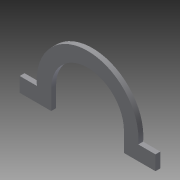
# Autodesk Inventor part: holder
Saved by Autodesk Inventor 2015 (Build 190159000, 159)
## iProperties
Created: 2014-08-30
Part Number: holder
Material: Generic
Document SubType Name: Modeling
Designer: shohei
Density: 1 g/cm^3
Appearance: Default
Author: shohei
Autodesk Inventor part; units mm, degrees
ref_plane "YZ Plane" through (0, 0, 0) normal (1, 0, 0) x (0, 1, 0)
ref_plane "XZ Plane" through (0, 0, 0) normal (0, 1, 0) x (-1, 0, 0)
ref_plane "XY Plane" through (0, 0, 0) normal (0, 0, 1) x (1, 0, 0)
sketch "Sketch1" plane through (0, 0, 0) normal (0, 1, 0) x (-1, 0, 0)
  arc A0 (104.5316, -9.9117) -> (-104.5321, -9.9065) centre (0, 0) ccw
  line L0 (104.5316, -9.9117) -> (140, -9.9117)
  line L1 (140, -9.9117) -> (140, -39.9117)
  line L2 (-140, -39.9117) -> (-140, -9.9065)
  line L3 (0, -68.8947) -> (0, 133.9861) projected
  line L4 (135.3627, -9.9117) -> (104.5316, -9.9117)
  line L5 (-104.5321, -9.9065) -> (-140, -9.9065)
  line L6 (74.3541, -9.8216) -> (74.3541, -9.9117)
  line L7 (74.3541, -9.8216) -> (74.3541, -9.9117)
  line L8 (140, -39.9117) -> (75, -39.9117)
  line L9 (-75, -39.9117) -> (-140, -39.9117)
  line L10 (-196, 0) -> (196, 0) projected
  arc A1 (74.3429, -9.9065) -> (74.3541, -9.8216) centre (0, 0) ccw
  arc A2 (75, 0) -> (-75, 0) centre (0, 0) ccw
  line L11 (75, 0) -> (75, -39.9117)
  line L12 (-75, -39.9117) -> (-75, 0)
  dimension "d3" = 30
  dimension "d4" = 280
  dimension "d5" = 140
  constraints: 22 end point, 9 perpendicular, 7 point on circle, 3 centre point, 3 point on line, 2 coincident, 2 horizontal, 1 parallel, 1 vertical
  measures "d3" distance of L0.end L1.end
  measures "d4" distance of L1.end L2.start
  measures "d5" distance between parallel lines of L1 L3
extrude "Extrusion2" add sketch "Sketch1" along normal blind 10 contours L0 L1 L8 L11 L10 A0 | L10 A2 L3 A0 | L3 A2 L10 A0 | L10 L12 L9 L2 L5 A0
body "Solid2"
